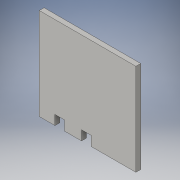
# Autodesk Inventor part: SideRWall
Saved by Autodesk Inventor 2016 (Build 200138000, 138)
## iProperties
Created: 2016-05-30
Part Number: SideRWall
Material: Generic
Document SubType Name: Modeling
Designer: cutrones
Density: 1 g/cm^3
Appearance: Default
Author: cutrones
Autodesk Inventor part; units mm, degrees
ref_plane "YZ Plane" through (0, 0, 0) normal (1, 0, 0) x (0, 1, 0)
ref_plane "XZ Plane" through (0, 0, 0) normal (0, 1, 0) x (-1, 0, 0)
ref_plane "XY Plane" through (0, 0, 0) normal (0, 0, 1) x (1, 0, 0)
sketch "Sketch1" plane through (0, 0, 0) normal (0, 0, 1) x (1, 0, 0)
  line L0 (0, 0) -> (254, 0)
  line L1 (254, 0) -> (254, 241.3)
  line L2 (254, 241.3) -> (0, 241.3)
  line L3 (0, 241.3) -> (0, 0)
  dimension "d0" = 254
  dimension "d1" = 241.3
  constraints: 8 end point, 2 parallel, 1 horizontal, 1 perpendicular
  measures "d0" distance of L1.end L2.end
  measures "d1" distance of L0.end L1.end
extrude "Extrusion1" add sketch "Sketch1" along normal mid plane 12.7
sketch "Sketch2" plane through (0, 0, 6.35) normal (0, 0, 1) x (1, 0, 0)
  line L0 (88.9, 244.858) -> (88.9, 0)
  line L1 (0, 241.3) -> (0, 0) projected
  line L2 (66.675, 127.7374) -> (88.9, 127.7374)
  line L3 (88.9, 83.4446) -> (111.125, 83.4446)
  line L4 (0, 0) -> (254, 0) projected
  line L5 (66.675, 25.4) -> (41.275, 25.4)
  line L6 (41.275, 25.4) -> (41.275, 0)
  line L7 (41.275, 0) -> (66.675, 0)
  line L8 (66.675, 0) -> (66.675, 25.4)
  line L9 (111.125, 25.4) -> (136.525, 25.4)
  line L10 (136.525, 25.4) -> (136.525, 0)
  line L11 (136.525, 0) -> (111.125, 0)
  line L12 (111.125, 0) -> (111.125, 25.4)
  dimension "d4" = 88.9
  dimension "d5" = 22.225
  dimension "d6" = 22.225
  dimension "d7" = 25.4
  dimension "d8" = 25.4
  dimension "d9" = 25.4
  dimension "d10" = 22.225
  dimension "d11" = 22.225
  constraints: 22 end point, 5 point on line, 4 parallel, 3 horizontal, 3 perpendicular, 1 vertical
  measures "d4" distance between parallel lines of L1 L0
  measures "d5" distance of L2.start L2.end
  measures "d6" distance of L3.start L3.end
  measures "d7" distance of L9.end L10.end
  measures "d8" distance between parallel lines of L10 L12
  measures "d9" distance of L5.start L5.end
  measures "d10" distance between parallel lines of L0 L8
  measures "d11" distance between parallel lines of L0 L12
extrude "Extrusion2" cut sketch "Sketch2" against normal through all
equation "\"d0\" = Width"
equation "\"d1\" = Height"
equation "\"Width\" = 254"
equation "\"Height\" = 241.3"
body "Solid1"
